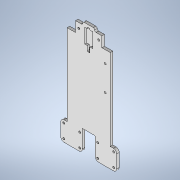
# Autodesk Inventor part: Основа робота
Saved by Autodesk Inventor 2020 (Build 240168000, 168)
## iProperties
Created: 2021-02-28
Part Number: Основа робота
Material: Типовые
Document SubType Name: Обычные детали
Designer: Антон
Density: 1 g/cm^3
Appearance: По умолчанию
Mass: 52.0111 g
Surface Area: 352.197 cm^2
Volume: 52.0111 cm^3
Sheet Metal Rule: По умолчанию
Author: Антон
Autodesk Inventor part; units mm, degrees
ref_plane "YZ Plane" through (0, 0, 0) normal (1, 0, 0) x (0, 1, 0)
ref_plane "XZ Plane" through (0, 0, 0) normal (0, 1, 0) x (-1, 0, 0)
ref_plane "XY Plane" through (0, 0, 0) normal (0, 0, 1) x (1, 0, 0)
sketch "Эскиз1" plane through (0, 0, 0) normal (0, 0, 1) x (1, 0, 0)
  line L0 (0, 0) -> (33.45, 0)
  line L1 (33.45, 0) -> (33.45, 172.55)
  line L2 (33.45, 172.55) -> (0, 172.55)
  line L3 (0, 172.55) -> (0, 0)
  line L4 (0, 0) -> (-9.9, 0)
  line L5 (-9.9, 0) -> (-9.9, 30.3)
  line L6 (-9.9, 30.3) -> (0, 30.3)
  line L7 (0, 30.3) -> (0, 0)
  line L8 (-9.9, 0) -> (-5.35, 0)
  line L9 (-5.35, 0) -> (-5.35, 4.55)
  line L10 (-5.35, 4.55) -> (-5.35, 25.75) construction
  circle A0 centre (-5.35, 25.75) radius 1.6
  circle A1 centre (-5.35, 4.55) radius 1.6
  line L11 (33.45, 0) -> (23.45, 0)
  line L12 (23.45, 0) -> (23.45, 33)
  line L13 (23.45, 33) -> (33.45, 33)
  line L14 (33.45, 33) -> (33.45, 0)
  line L15 (23.45, 4.55) -> (19.45, 4.55)
  line L16 (23.45, 25.75) -> (19.45, 25.75)
  circle A2 centre (19.45, 25.75) radius 1.6
  circle A3 centre (19.45, 4.55) radius 1.6
  line L17 (33.45, 172.55) -> (33.45, 172.55)
  line L18 (33.45, 172.55) -> (18, 172.55)
  line L19 (19.45, 25.75) -> (19.45, 4.55) construction
  circle A4 centre (17.95, 164.55) radius 1.6
  line L20 (13, 172.55) -> (13, 156.55)
  line L21 (13, 156.55) -> (0, 156.55)
  line L22 (0, 156.55) -> (0, 129.6)
  line L23 (33.45, 172.55) -> (24.2, 172.55)
  line L24 (24.2, 172.55) -> (24.2, 177)
  line L25 (24.2, 177) -> (33.45, 177)
  line L26 (33.45, 177) -> (33.45, 172.55)
  line L27 (0.5313, 124.1884) -> (4, 120.7198)
  line L28 (4, 120.7198) -> (4, 143.125)
  line L29 (4, 143.125) -> (0, 139.125)
  point P0 (0, 30.3)
  point P1 (0, 182.1)
  point P2 (19.45, 15.15)
  point P3 (-5.35, 15.15)
  point P4 (0, 156.55)
  point P5 (13, 164.55)
  point P6 (0, 125.55)
  dimension "d0" = 33.45
  dimension "d1" = 172.55
  dimension "d191" = 9.9
  dimension "d192" = 30.3
  dimension "d207" = 4.55
  dimension "d208" = 4.55
  dimension "d209" = 21.2
  dimension "d210" = 10
  dimension "d211" = 33
  dimension "d215" = 4
  dimension "d290" = 3.2
  dimension "d387" = 21.2
  dimension "d418" = 4.55
  dimension "d421" = 3.2
  dimension "d427" = 13
  dimension "d428" = 16
  dimension "d433" = 4.95
  dimension "d448" = 9.25
  dimension "d450" = 4.45
  dimension "d453" = 45
  dimension "d454" = 4
  dimension "d455" = 17.425
  constraints: 60 end point, 10 parallel, 8 perpendicular, 8 point on line, 6 horizontal, 5 centre point, 4 coincident, 3 equal radius, 3 midpoint, 2 collinear, 2 horizontal alignment, 2 vertical
  measures "d0" distance of L2.end L1.end
  measures "d1" distance of L1.end L0.end
  measures "d191" distance of L5.end L6.end
  measures "d192" distance of L4.end L5.end
  measures "d207" distance of L4.end L8.end
  measures "d208" distance of L8.end L9.end
  measures "d209" distance of L9.end L10.end
  measures "d210" distance of L12.end L13.end
  measures "d211" distance of L11.end L12.end
  measures "d215" distance of L16.start L16.end
  measures "d290" diameter of A2
  measures "d387" distance of L19.end L19.start
  measures "d418" distance from line of L0 L15.end
  measures "d421" diameter of A4
  measures "d427" distance of L20.end L21.end
  measures "d428" distance of L20.start L20.end
  measures "d433" distance of A4.centre point (13, 164.55)
  measures "d448" distance of L24.end L25.end
  measures "d450" distance of L23.end L24.end
  measures "d453" angle of L3 L29
  measures "d454" distance between parallel lines of L3 L28
  measures "d455" distance of L21.end L29.end
extrude "Выдавливание1" add sketch "Эскиз1" along normal blind 4 contours L3 L21 L20 L2 L1 L13 L12 L0 | L4 L5 L6 L3 | L2 L24 L25 L26
mirror "Зеркальное отражение1" about plane through (33.45, 33, 0) normal (1, 0, 0)
sketch "Эскиз32" plane through (0, 0, 4) normal (0, 0, 1) x (1, 0, 0)
  line L0 (23.45, 33) -> (43.45, 33) construction
  line L1 (33.45, 33) -> (33.45, 118.2) construction
  line L2 (33.45, 118.2) -> (58.9, 118.2) construction
  line L3 (58.9, 137.7) -> (58.9, 98.7) construction
  dimension "d474" = 39
  dimension "d475" = 25.45
  dimension "d476" = 85.2
  constraints: 6 end point, 2 midpoint, 1 horizontal, 1 perpendicular, 1 vertical
  measures "d474" distance of L3.start L3.end
  measures "d475" distance of L1.end L2.end
  measures "d476" distance of L1.start L1.end
hole "Отверстие14" at (58.9, 137.7, 4) at (58.9, 98.7, 4) direction (0, 0, -1) diameter 3.2 end through all
sketch "Эскиз33" plane through (0, 0, 4) normal (0, 0, 1) x (1, 0, 0)
  line L0 (24.2, 177) -> (33.45, 177) construction
  line L1 (33.45, 177) -> (33.45, 173) construction
  line L2 (39.7, 171) -> (27.2, 171)
  line L3 (27.2, 171) -> (27.2, 148.2)
  line L4 (27.2, 148.2) -> (39.7, 148.2)
  line L5 (39.7, 148.2) -> (39.7, 171)
  line L6 (31.45, 173) -> (35.45, 173)
  line L7 (35.45, 173) -> (35.45, 171)
  line L8 (35.45, 171) -> (31.45, 171)
  line L9 (31.45, 171) -> (31.45, 173)
  line L10 (31.45, 148.2) -> (35.45, 148.2)
  line L11 (35.45, 148.2) -> (35.45, 140.2)
  line L12 (35.45, 140.2) -> (31.45, 140.2)
  line L13 (31.45, 140.2) -> (31.45, 148.2)
  point P0 (0, 0)
  point P1 (42.7, 177)
  point P2 (33.45, 171)
  point P3 (33.45, 148.2)
  point P4 (31.45, 171)
  dimension "d465" = 12.5
  dimension "d466" = 22.8
  dimension "d467" = 2
  dimension "d468" = 4
  dimension "d469" = 4
  dimension "d470" = 4
  dimension "d471" = 8
  constraints: 27 end point, 6 parallel, 5 midpoint, 3 horizontal, 3 perpendicular, 1 vertical
  measures "d465" distance between parallel lines of L5 L3
  measures "d466" distance of L4.end L2.start
  measures "d467" distance of L6.end L7.end
  measures "d468" distance of L6.start L6.end
  measures "d469" distance of L0.end L1.end
  measures "d470" distance of L11.end L12.end
  measures "d471" distance of L10.end L11.end
extrude "Выдавливание14" cut sketch "Эскиз33" against normal blind 3
fillet "Сопряжение14" radius 1 2 edges at (35.45, 140.2, 2.5) (31.45, 140.2, 2.5)
fillet "Сопряжение13" radius 2.225 4 edges at (24.2, 172.55, 2) (24.2, 177, 2) (42.7, 172.55, 2) (42.7, 177, 2)
fillet "Сопряжение2" radius 5.05 6 edges at (-9.9, 30.3, 2) (-9.9, 0, 2) (23.45, 0, 2) (43.45, 0, 2) (76.8, 0, 2) (76.8, 30.3, 2)
sketch "Эскиз19" plane through (0, 0, 0) normal (0, 0, -1) x (-1, 0, 0)
  line L0 (-24.2, 172.55) -> (-13, 172.55) projected
  line L1 (-20.75, 166.1666) -> (-17.95, 167.7832)
  line L2 (-17.95, 167.7832) -> (-15.15, 166.1666)
  line L3 (-15.15, 166.1666) -> (-15.15, 162.9334)
  line L4 (-15.15, 162.9334) -> (-17.95, 161.3168)
  line L5 (-17.95, 161.3168) -> (-20.75, 162.9334)
  line L6 (-20.75, 162.9334) -> (-20.75, 166.1666)
  line L7 (0, 156.55) -> (0, 30.3) projected
  circle A0 centre (-17.95, 164.55) radius 1.6 projected
  point P0 (0, 139.6)
  point P1 (-78, 139.6)
  point P2 (-14, 129.6)
  point P3 (-64, 129.6)
  point P4 (0, 119.25)
  point P5 (0, 129.6)
  point P6 (-78, 129.6)
  point P7 (-53.9, 172.55)
  point P8 (0, 107.125)
  point P9 (-33.45, 140.55)
  dimension "d423" = 5.6
  constraints: 12 end point, 1 coincident, 1 parallel, 14 other
  measures "d423" distance between parallel lines of L3 L6
extrude "Выдавливание7" cut sketch "Эскиз19" against normal blind 2.6 contours L1 L2 L3 L4 L5 L6 | A0
fillet "Сопряжение12" [suppressed]
sketch "Эскиз25" plane through (0, 0, 0) normal (0, 0, -1) x (-1, 0, 0)
  circle A0 centre (-19.45, 25.75) radius 1.6 projected
  circle A1 centre (-19.45, 4.55) radius 1.6 projected
  circle A2 centre (5.35, 25.75) radius 1.6 projected
  circle A3 centre (5.35, 4.55) radius 1.6 projected
  circle A4 centre (-47.45, 25.75) radius 1.6 projected
  circle A5 centre (-47.45, 4.55) radius 1.6 projected
  circle A6 centre (-72.25, 4.55) radius 1.6 projected
  circle A7 centre (-72.25, 25.75) radius 1.6 projected
  circle A8 centre (-48.95, 164.55) radius 1.6 projected
  circle A9 centre (-48.95, 164.55) radius 1.6 projected
  point P0 (0, 0)
  constraints: 9 coincident
pattern_sketch "Массив по эскизу1" of "Выдавливание7" from (17.95, 164.55, 0) copies at (19.45, 25.75, 0) at (19.45, 4.55, 0) at (-5.35, 25.75, 0) at (-5.35, 4.55, 0) at (47.45, 25.75, 0) at (47.45, 4.55, 0) at (72.25, 4.55, 0) at (72.25, 25.75, 0) at (48.95, 164.55, 0)
fillet "Сопряжение11" [suppressed]
sketch "Эскиз31" plane through (0, 0, 0) normal (0, 0, -1) x (-1, 0, 0)
  line L0 (-66.9, 124.55) -> (0, 124.55) construction
  line L1 (0, 156.55) -> (0, 33) construction
  line L2 (0, 33) -> (-66.9, 33) construction
  line L3 (-66.9, 33) -> (-66.9, 124.55) construction
  line L4 (-53.9, 156.55) -> (-66.9, 156.55) projected
  line L5 (-66.9, 156.55) -> (-66.9, 30.3) projected
  line L6 (0, 156.55) -> (0, 30.3) projected
  line L7 (-23.45, 33) -> (-43.45, 33) projected
  line L8 (-42.4647, 94.2344) -> (-43.1267, 99.208)
  line L9 (-43.1267, 99.208) -> (-42.0742, 99.7114)
  line L10 (-42.0742, 99.7114) -> (-41.4245, 93.2602)
  line L11 (-41.4245, 93.2602) -> (-42.35, 92.8176)
  line L12 (-42.35, 92.8176) -> (-46.9556, 97.3765)
  line L13 (-46.9556, 97.3765) -> (-45.9076, 97.8778)
  line L14 (-45.9076, 97.8778) -> (-42.4647, 94.2344)
  line L15 (-37.9359, 94.9289) -> (-38.8523, 94.4906)
  line L16 (-38.8523, 94.4906) -> (-40.8074, 98.5781)
  line L17 (-40.8074, 98.5781) -> (-39.891, 99.0164)
  line L18 (-39.891, 99.0164) -> (-37.9359, 94.9289)
  spline S0 degree 2 poles (-41.3742, 99.6114) (-41.474, 99.8201) (-41.3409, 100.2294) (-40.8418, 100.4681) (-40.4351, 100.317) (-40.3353, 100.1083) knots 0 0 0 1 2 3 4 4 4
  spline S1 degree 2 poles (-40.3353, 100.1083) (-40.2355, 99.8997) (-40.3753, 99.4927) (-40.8743, 99.254) (-41.2743, 99.4027) (-41.3742, 99.6114) knots 0 0 0 1 2 3 4 4 4
  spline S2 degree 2 poles (-38.1017, 97.4083) (-38.3881, 98.0072) (-38.374, 99.2013) (-37.7594, 100.1308) (-37.2014, 100.3977) knots 0 0 0 1 2 3 3 3
  spline S3 degree 2 poles (-37.2014, 100.3977) (-36.3758, 100.7926) (-34.8315, 100.2213) (-34.3697, 99.3607) knots 0 0 0 1 2 2 2
  line L19 (-34.3697, 99.3607) -> (-34.261, 99.1451)
  spline S4 degree 2 poles (-34.261, 99.1451) (-33.9724, 98.5417) (-33.9839, 97.3655) (-34.6009, 96.4294) (-35.1634, 96.1603) knots 0 0 0 1 2 3 3 3
  spline S5 degree 2 poles (-35.1634, 96.1603) (-36.0299, 95.7458) (-37.62, 96.4012) (-38.08, 97.363) knots 0 0 0 1 2 2 2
  line L20 (-38.08, 97.363) -> (-38.1017, 97.4083)
  spline S6 degree 2 poles (-37.1484, 97.7695) (-36.8468, 97.139) (-35.9822, 96.6717) (-35.0522, 97.1166) (-34.8823, 98.0898) (-35.2164, 98.7884) knots 0 0 0 1 2 3 4 4 4
  spline S7 degree 2 poles (-35.2164, 98.7884) (-35.5137, 99.4099) (-36.3917, 99.8819) (-36.8499, 99.6627) knots 0 0 0 1 2 2 2
  spline S8 degree 2 poles (-36.8499, 99.6627) (-37.299, 99.4479) (-37.4869, 98.4772) (-37.1484, 97.7695) knots 0 0 0 1 2 2 2
  line L21 (-31.5529, 97.9821) -> (-32.4693, 97.5437)
  line L22 (-32.4693, 97.5437) -> (-35.2468, 103.3506)
  line L23 (-35.2468, 103.3506) -> (-34.3305, 103.7889)
  line L24 (-34.3305, 103.7889) -> (-31.5529, 97.9821)
  spline S9 degree 2 poles (-28.7169, 99.2438) (-29.588, 98.8272) (-31.1995, 99.411) (-31.6357, 100.3228) knots 0 0 0 1 2 2 2
  line L25 (-31.6357, 100.3228) -> (-31.6899, 100.4362)
  spline S10 degree 2 poles (-31.6899, 100.4362) (-31.9829, 101.0487) (-31.9733, 102.2406) (-31.3764, 103.1839) (-30.8502, 103.4356) knots 0 0 0 1 2 3 3 3
  spline S11 degree 2 poles (-30.8502, 103.4356) (-30.0155, 103.8349) (-28.5937, 103.205) (-28.1293, 102.2341) knots 0 0 0 1 2 2 2
  line L26 (-28.1293, 102.2341) -> (-27.9514, 101.8621)
  line L27 (-27.9514, 101.8621) -> (-30.6234, 100.584)
  spline S12 degree 2 poles (-30.6234, 100.584) (-30.3395, 100.0955) (-29.4632, 99.79) (-29.014, 100.0048) knots 0 0 0 1 2 2 2
  spline S13 degree 2 poles (-29.014, 100.0048) (-28.3834, 100.3064) (-28.2273, 101.0055) knots 0 0 0 1 1 1
  line L28 (-28.2273, 101.0055) -> (-27.5071, 100.7702)
  spline S14 degree 2 poles (-27.5071, 100.7702) (-27.5763, 100.2855) (-28.2043, 99.489) (-28.7169, 99.2438) knots 0 0 0 1 2 2 2
  spline S15 degree 2 poles (-30.5032, 102.6985) (-30.8797, 102.5184) (-31.0931, 101.7641) (-30.931, 101.2619) knots 0 0 0 1 2 2 2
  line L29 (-30.931, 101.2619) -> (-29.1798, 102.0996)
  line L30 (-29.1798, 102.0996) -> (-29.2124, 102.1676)
  spline S16 degree 2 poles (-29.2124, 102.1676) (-29.4655, 102.6151) (-30.1221, 102.8808) (-30.5032, 102.6985) knots 0 0 0 1 2 2 2
  line L31 (-27.6819, 106.0771) -> (-27.2067, 105.0836)
  line L32 (-27.2067, 105.0836) -> (-26.4854, 105.4286)
  line L33 (-26.4854, 105.4286) -> (-26.1599, 104.7482)
  line L34 (-26.1599, 104.7482) -> (-26.8812, 104.4031)
  line L35 (-26.8812, 104.4031) -> (-25.7897, 102.1212)
  spline S17 degree 2 poles (-25.7897, 102.1212) (-25.6769, 101.8853) (-25.3911, 101.7656) (-25.1552, 101.8785) knots 0 0 0 1 2 2 2
  spline S18 degree 2 poles (-25.1552, 101.8785) (-24.9964, 101.9544) (-24.8504, 102.0688) knots 0 0 0 1 1 1
  line L36 (-24.8504, 102.0688) -> (-24.5119, 101.3611)
  spline S19 degree 2 poles (-24.5119, 101.3611) (-24.7837, 101.1252) (-25.0741, 100.9863) knots 0 0 0 1 1 1
  spline S20 degree 2 poles (-25.0741, 100.9863) (-26.1311, 100.4807) (-26.6888, 101.6466) knots 0 0 0 1 1 1
  line L37 (-26.6888, 101.6466) -> (-27.7976, 103.9648)
  line L38 (-27.7976, 103.9648) -> (-28.469, 103.6436)
  line L39 (-28.469, 103.6436) -> (-28.7945, 104.3241)
  line L40 (-28.7945, 104.3241) -> (-28.1231, 104.6453)
  line L41 (-28.1231, 104.6453) -> (-28.5983, 105.6388)
  line L42 (-28.5983, 105.6388) -> (-27.6819, 106.0771)
  line L43 (-41.6745, 88.218) -> (-38.0732, 84.7563)
  line L44 (-38.0732, 84.7563) -> (-38.508, 89.7327)
  line L45 (-38.508, 89.7327) -> (-37.2695, 90.3251)
  line L46 (-37.2695, 90.3251) -> (-34.6373, 84.8222)
  line L47 (-34.6373, 84.8222) -> (-35.59, 84.3665)
  line L48 (-35.59, 84.3665) -> (-36.458, 86.1811)
  line L49 (-36.458, 86.1811) -> (-37.5237, 88.6538)
  line L50 (-37.5237, 88.6538) -> (-37.1189, 83.6352)
  line L51 (-37.1189, 83.6352) -> (-37.8039, 83.3075)
  line L52 (-37.8039, 83.3075) -> (-41.4547, 86.7679)
  line L53 (-41.4547, 86.7679) -> (-40.2007, 84.3909)
  line L54 (-40.2007, 84.3909) -> (-39.3327, 82.5763)
  line L55 (-39.3327, 82.5763) -> (-40.2854, 82.1206)
  line L56 (-40.2854, 82.1206) -> (-42.9176, 87.6235)
  line L57 (-42.9176, 87.6235) -> (-41.6745, 88.218)
  line L58 (-33.1023, 87.7082) -> (-33.311, 87.0955)
  line L59 (-33.311, 87.0955) -> (-32.673, 85.7618)
  line L60 (-32.673, 85.7618) -> (-33.5939, 85.3213)
  line L61 (-33.5939, 85.3213) -> (-36.3715, 91.1281)
  line L62 (-36.3715, 91.1281) -> (-35.4506, 91.5686)
  line L63 (-35.4506, 91.5686) -> (-33.847, 88.2161)
  line L64 (-33.847, 88.2161) -> (-33.7326, 88.7112)
  line L65 (-33.7326, 88.7112) -> (-33.2127, 90.5263)
  line L66 (-33.2127, 90.5263) -> (-32.1103, 91.0536)
  line L67 (-32.1103, 91.0536) -> (-32.8142, 88.6209)
  line L68 (-32.8142, 88.6209) -> (-29.9919, 87.0442)
  line L69 (-29.9919, 87.0442) -> (-31.0534, 86.5365)
  line L70 (-31.0534, 86.5365) -> (-33.1023, 87.7082)
  spline S21 degree 2 poles (-29.447, 88.4923) (-29.1929, 88.6138) (-28.7728, 88.458) (-28.6686, 88.2402) knots 0 0 0 1 2 2 2
  spline S22 degree 2 poles (-28.6686, 88.2402) (-28.5644, 88.0225) (-28.7112, 87.6066) (-28.9652, 87.4851) knots 0 0 0 1 2 2 2
  spline S23 degree 2 poles (-28.9652, 87.4851) (-29.2102, 87.368) (-29.6351, 87.5103) (-29.8434, 87.9459) (-29.701, 88.3707) (-29.447, 88.4923) knots 0 0 0 1 2 3 4 4 4
  line L71 (-24.371, 89.7328) -> (-25.3237, 89.2771)
  line L72 (-25.3237, 89.2771) -> (-27.9559, 94.78)
  line L73 (-27.9559, 94.78) -> (-27.0032, 95.2357)
  line L74 (-27.0032, 95.2357) -> (-24.371, 89.7328)
  line L75 (-21.8318, 92.4191) -> (-22.4938, 97.3926)
  line L76 (-22.4938, 97.3926) -> (-21.4414, 97.8961)
  line L77 (-21.4414, 97.8961) -> (-20.7917, 91.4449)
  line L78 (-20.7917, 91.4449) -> (-21.7171, 91.0022)
  line L79 (-21.7171, 91.0022) -> (-26.3227, 95.5612)
  line L80 (-26.3227, 95.5612) -> (-25.2748, 96.0625)
  line L81 (-25.2748, 96.0625) -> (-21.8318, 92.4191)
  point P0 (0, 0)
  point P1 (-69, 97.45)
  point P2 (-69, 32.99)
  point P3 (0, 97.45)
  point P4 (-33.45, 33)
  point P5 (-66.9, 30.3)
  point P6 (0, 107.125)
  point P7 (-66.9, 107.125)
  constraints: 2 collinear, 1 horizontal, 1 vertical, 4 other
emboss "Рельеф1" sketch "Эскиз31" operation cut depth 0.5 direction (0, 0, 1)
equation "\"d130\" = 5.6"
equation "\"Радиус_гибки\" = Толщина"
equation "\"Ширина_просечки\" = Толщина"
equation "\"Глубина_просечки\" = 0.5 * Толщина"
equation "\"Размер_просечки\" = 4 * Толщина"
equation "\"Мин_остаток\" = 2 * Толщина"
equation "\"Радиус_перехода\" = Радиус_гибки"
equation "\"Радиус_Якоби\" = Толщина"
equation "\"Размер_зазора\" = Толщина"
equation "\"Гайка_М3_з\" = 5.6"
equation "\"Толщина\" = 0.5"
